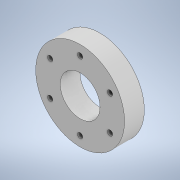
# Autodesk Inventor part: IndexerWheelSpacer
Saved by Autodesk Inventor 2020 (Build 240168000, 168)
## iProperties
Created: 2020-01-26
Part Number: IndexerWheelSpacer
Material: Generic
Document SubType Name: Modeling
Designer: srini
Density: 1 g/cm^3
Appearance: Default
Author: srini
Autodesk Inventor part; units mm, degrees
ref_plane "YZ Plane" through (0, 0, 0) normal (1, 0, 0) x (0, 1, 0)
ref_plane "XZ Plane" through (0, 0, 0) normal (0, 1, 0) x (-1, 0, 0)
ref_plane "XY Plane" through (0, 0, 0) normal (0, 0, 1) x (1, 0, 0)
sketch "Sketch1" plane through (0, 0, 0) normal (0, 0, 1) x (1, 0, 0)
  circle A0 centre (0, 0) radius 25.6
  circle A1 centre (0, 44.45) radius 3.3734
  circle A2 centre (-38.4948, 22.225) radius 3.3734
  circle A3 centre (-38.4948, -22.225) radius 3.3734
  circle A4 centre (0, -44.45) radius 3.3734
  circle A5 centre (38.4948, -22.225) radius 3.3734
  circle A6 centre (38.4948, 22.225) radius 3.3734
  circle A7 centre (0, 0) radius 57.15
  dimension "d0" = 51.2
  dimension "d1" = 44.45
  dimension "d2" = 6.7469
  dimension "d5" = 360
  dimension "d7" = 114.3
  constraints: 8 centre point, 2 coincident, 1 vertical alignment, 13 other
  measures "d0" diameter of A0
  measures "d1" distance of point (0, 0) A1.centre
  measures "d2" diameter of A1
  measures "d7" diameter of A7
extrude "Extrusion1" add sketch "Sketch1" along normal blind 25.4
body "Solid1"
